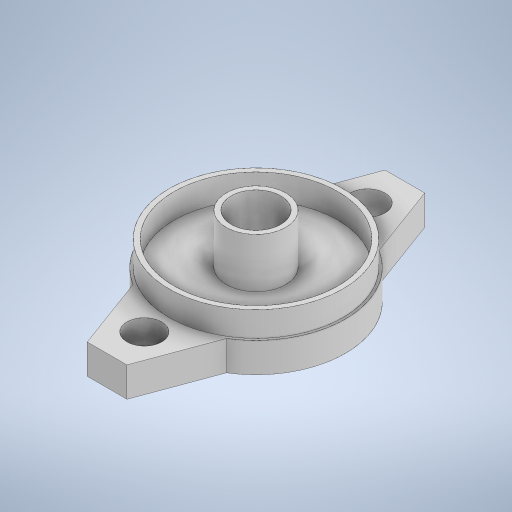
# Autodesk Inventor part: Chumacera con rodamiento 10 mm kfl000
Saved by Autodesk Inventor 2024 (Build 280153000, 153)
## iProperties
Created: 2024-04-26
Part Number: Chumacera con rodamiento 10 mm kfl000
Material: Genérico
Document SubType Name: Modeling
Designer: alexa
Density: 1 g/cm^3
Appearance: Valor por defecto
Author: alexa
Autodesk Inventor part; units mm, degrees
ref_plane "YZ Plane" through (0, 0, 0) normal (1, 0, 0) x (0, 1, 0)
ref_plane "XZ Plane" through (0, 0, 0) normal (0, 1, 0) x (-1, 0, 0)
sketch "Sketch1" plane through (0, 0, 0) normal (0, 1, 0) x (-1, 0, 0)
  circle A0 centre (0, 22.5) radius 3.5
  line L0 (0, 30) -> (4, 30)
  line L1 (4, 30) -> (9.4194, 15.3387)
  line L2 (0, 30) -> (-4, 30)
  line L3 (-4, 30) -> (-9.4194, 15.3387)
  circle A1 centre (0, -22.5) radius 3.5
  line L4 (0, -30) -> (4, -30)
  line L5 (4, -30) -> (9.4194, -15.3387)
  line L6 (0, -30) -> (-4, -30)
  line L7 (-4, -30) -> (-9.4194, -15.3387)
  arc A2 (-9.4194, 15.3387) -> (-9.4194, -15.3387) centre (0, 0) ccw
  arc A3 (9.4194, -15.3387) -> (9.4194, 15.3387) centre (0, 0) ccw
  constraints: 16 end point, 4 centre point, 4 point on circle, 1 coincident, 1 horizontal
extrude "Extrusion1" add sketch "Sketch1" along normal blind 6
ref_plane "Work Plane1" through (0, 6, 0) normal (0, 1, 0) x (1, 0, 0)
sketch "Sketch2" plane through (0, 6, 0) normal (0, 1, 0) x (1, 0, 0)
  circle A0 centre (0, 0) radius 17.5
  circle A1 centre (0, 0) radius 16.5
  dimension "d9" = 35
  dimension "d12" = 33
  constraints: 2 centre point, 1 coincident
  measures "d9" diameter of A0
  measures "d12" diameter of A1
extrude "Extrusion2" add sketch "Sketch2" along normal blind 5
sketch "Sketch3" plane through (0, 6, 0) normal (0, 1, 0) x (1, 0, 0)
  circle A0 centre (0, 0) radius 5
  circle A1 centre (0, 0) radius 6
  dimension "d15" = 10
  dimension "d16" = 12
  constraints: 2 centre point, 2 coincident
  measures "d15" diameter of A0
  measures "d16" diameter of A1
extrude "Extrusion3" add sketch "Sketch3" along normal blind 10
body "Solid1"
